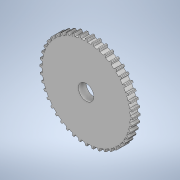
# Autodesk Inventor part: Part14
Saved by Autodesk Inventor 2021 (Build 250183000, 183)
## iProperties
Created: 2022-12-09
Part Number: Part14
Material: Generic
Document SubType Name: Modeling
Designer: user
Density: 1 g/cm^3
Appearance: Default
Author: user
Autodesk Inventor part; units mm, degrees
ref_plane "YZ Plane" through (0, 0, 0) normal (1, 0, 0) x (0, 1, 0)
ref_plane "XZ Plane" through (0, 0, 0) normal (0, 1, 0) x (-1, 0, 0)
ref_plane "XY Plane" through (0, 0, 0) normal (0, 0, 1) x (1, 0, 0)
sketch "Sketch1" plane through (0, 0, 0) normal (0, 0, 1) x (1, 0, 0)
  circle A0 centre (0, 0) radius 20
  arc A1 (-3.5207, 113.9456) -> (-12.7313, 113.2869) centre (0, 0) ccw
  arc A2 (12.7313, 113.2869) -> (3.5207, 113.9456) centre (0, 0) ccw
  arc A3 (-19.701, 112.2848) -> (-28.7241, 110.3219) centre (0, 0) ccw
  arc A4 (-35.4803, 108.3381) -> (-44.1322, 105.1111) centre (0, 0) ccw
  arc A5 (28.7241, 110.3219) -> (19.701, 112.2848) centre (0, 0) ccw
  arc A6 (44.1322, 105.1111) -> (35.4803, 108.3381) centre (0, 0) ccw
  arc A7 (58.6419, 97.7606) -> (50.5373, 102.186) centre (0, 0) ccw
  arc A8 (-50.5373, 102.186) -> (-58.6419, 97.7606) centre (0, 0) ccw
  arc A9 (-64.5655, 93.9537) -> (-71.9577, 88.4199) centre (0, 0) ccw
  arc A10 (-77.2793, 83.8088) -> (-83.8088, 77.2793) centre (0, 0) ccw
  arc A11 (-88.4199, 71.9577) -> (-93.9537, 64.5655) centre (0, 0) ccw
  arc A12 (-97.7606, 58.6419) -> (-102.186, 50.5373) centre (0, 0) ccw
  arc A13 (-105.1111, 44.1322) -> (-108.3381, 35.4803) centre (0, 0) ccw
  arc A14 (-110.3219, 28.7241) -> (-112.2848, 19.701) centre (0, 0) ccw
  arc A15 (-113.2869, 12.7313) -> (-113.9456, 3.5207) centre (0, 0) ccw
  arc A16 (-113.9456, -3.5207) -> (-113.2869, -12.7313) centre (0, 0) ccw
  arc A17 (-112.2848, -19.701) -> (-110.3219, -28.7241) centre (0, 0) ccw
  arc A18 (-108.3381, -35.4803) -> (-105.1111, -44.1322) centre (0, 0) ccw
  arc A19 (-102.186, -50.5373) -> (-97.7606, -58.6419) centre (0, 0) ccw
  arc A20 (-93.9537, -64.5655) -> (-88.4199, -71.9577) centre (0, 0) ccw
  arc A21 (-83.8088, -77.2793) -> (-77.2793, -83.8088) centre (0, 0) ccw
  arc A22 (-71.9577, -88.4199) -> (-64.5655, -93.9537) centre (0, 0) ccw
  arc A23 (-58.6419, -97.7606) -> (-50.5373, -102.186) centre (0, 0) ccw
  arc A24 (-44.1322, -105.1111) -> (-35.4803, -108.3381) centre (0, 0) ccw
  arc A25 (-28.7241, -110.3219) -> (-19.701, -112.2848) centre (0, 0) ccw
  arc A26 (-12.7313, -113.2869) -> (-3.5207, -113.9456) centre (0, 0) ccw
  arc A27 (3.5207, -113.9456) -> (12.7313, -113.2869) centre (0, 0) ccw
  arc A28 (19.701, -112.2848) -> (28.7241, -110.3219) centre (0, 0) ccw
  arc A29 (35.4803, -108.3381) -> (44.1322, -105.1111) centre (0, 0) ccw
  arc A30 (50.5373, -102.186) -> (58.6419, -97.7606) centre (0, 0) ccw
  arc A31 (64.5655, -93.9537) -> (71.9577, -88.4199) centre (0, 0) ccw
  arc A32 (77.2793, -83.8088) -> (83.8088, -77.2793) centre (0, 0) ccw
  arc A33 (88.4199, -71.9577) -> (93.9537, -64.5655) centre (0, 0) ccw
  arc A34 (97.7606, -58.6419) -> (102.186, -50.5373) centre (0, 0) ccw
  arc A35 (105.1111, -44.1322) -> (108.3381, -35.4803) centre (0, 0) ccw
  arc A36 (110.3219, -28.7241) -> (112.2848, -19.701) centre (0, 0) ccw
  arc A37 (113.2869, -12.7313) -> (113.9456, -3.5207) centre (0, 0) ccw
  arc A38 (113.9456, 3.5207) -> (113.2869, 12.7313) centre (0, 0) ccw
  arc A39 (112.2848, 19.701) -> (110.3219, 28.7241) centre (0, 0) ccw
  arc A40 (108.3381, 35.4803) -> (105.1111, 44.1322) centre (0, 0) ccw
  arc A41 (102.186, 50.5373) -> (97.7606, 58.6419) centre (0, 0) ccw
  arc A42 (93.9537, 64.5655) -> (88.4199, 71.9577) centre (0, 0) ccw
  arc A43 (83.8088, 77.2793) -> (77.2793, 83.8088) centre (0, 0) ccw
  arc A44 (71.9577, 88.4199) -> (64.5655, 93.9537) centre (0, 0) ccw
  line L0 (-3.5207, 113.9456) -> (-2.1115, 119.9814)
  line L1 (-2.1115, 119.9814) -> (0, 120)
  line L2 (0, 120) -> (2.1115, 119.9814)
  line L3 (2.1115, 119.9814) -> (3.5207, 113.9456)
  line L4 (-19.701, 112.2848) -> (-19.1651, 118.4597)
  line L5 (-19.1651, 118.4597) -> (-17.0778, 118.7786)
  line L6 (-17.0778, 118.7786) -> (-14.9851, 119.0607)
  line L7 (-14.9851, 119.0607) -> (-12.7313, 113.2869)
  line L8 (-35.4803, 108.3381) -> (-35.8286, 114.5265)
  line L9 (-35.8286, 114.5265) -> (-33.8079, 115.1392)
  line L10 (-33.8079, 115.1392) -> (-31.7767, 115.7162)
  line L11 (-31.7767, 115.7162) -> (-28.7241, 110.3219)
  line L12 (-50.5373, 102.186) -> (-51.7628, 108.2618)
  line L13 (-51.7628, 108.2618) -> (-49.8498, 109.1558)
  line L14 (-49.8498, 109.1558) -> (-47.9214, 110.0161)
  line L15 (-47.9214, 110.0161) -> (-44.1322, 105.1111)
  line L16 (-64.5655, 93.9537) -> (-66.6432, 99.7932)
  line L17 (-66.6432, 99.7932) -> (-64.8769, 100.9504)
  line L18 (-64.8769, 100.9504) -> (-63.0905, 102.0764)
  line L19 (-63.0905, 102.0764) -> (-58.6419, 97.7606)
  line L20 (-77.2793, 83.8088) -> (-80.1669, 89.2932)
  line L21 (-80.1669, 89.2932) -> (-78.5833, 90.6899)
  line L22 (-78.5833, 90.6899) -> (-76.9754, 92.0586)
  line L23 (-76.9754, 92.0586) -> (-71.9577, 88.4199)
  line L24 (-88.4199, 71.9577) -> (-92.0586, 76.9754)
  line L25 (-92.0586, 76.9754) -> (-90.6899, 78.5833)
  line L26 (-90.6899, 78.5833) -> (-89.2932, 80.1669)
  line L27 (-89.2932, 80.1669) -> (-83.8088, 77.2793)
  line L28 (-97.7606, 58.6419) -> (-102.0764, 63.0905)
  line L29 (-102.0764, 63.0905) -> (-100.9504, 64.8769)
  line L30 (-100.9504, 64.8769) -> (-99.7932, 66.6432)
  line L31 (-99.7932, 66.6432) -> (-93.9537, 64.5655)
  line L32 (-105.1111, 44.1322) -> (-110.0161, 47.9214)
  line L33 (-110.0161, 47.9214) -> (-109.1558, 49.8498)
  line L34 (-109.1558, 49.8498) -> (-108.2618, 51.7628)
  line L35 (-108.2618, 51.7628) -> (-102.186, 50.5373)
  line L36 (-110.3219, 28.7241) -> (-115.7162, 31.7767)
  line L37 (-115.7162, 31.7767) -> (-115.1392, 33.8079)
  line L38 (-115.1392, 33.8079) -> (-114.5265, 35.8286)
  line L39 (-114.5265, 35.8286) -> (-108.3381, 35.4803)
  line L40 (-113.2869, 12.7313) -> (-119.0607, 14.9851)
  line L41 (-119.0607, 14.9851) -> (-118.7786, 17.0778)
  line L42 (-118.7786, 17.0778) -> (-118.4597, 19.1651)
  line L43 (-118.4597, 19.1651) -> (-112.2848, 19.701)
  line L44 (-113.9456, -3.5207) -> (-119.9814, -2.1115)
  line L45 (-119.9814, -2.1115) -> (-120, 0)
  line L46 (-120, 0) -> (-119.9814, 2.1115)
  line L47 (-119.9814, 2.1115) -> (-113.9456, 3.5207)
  line L48 (-112.2848, -19.701) -> (-118.4597, -19.1651)
  line L49 (-118.4597, -19.1651) -> (-118.7786, -17.0778)
  line L50 (-118.7786, -17.0778) -> (-119.0607, -14.9851)
  line L51 (-119.0607, -14.9851) -> (-113.2869, -12.7313)
  line L52 (-108.3381, -35.4803) -> (-114.5265, -35.8286)
  line L53 (-114.5265, -35.8286) -> (-115.1392, -33.8079)
  line L54 (-115.1392, -33.8079) -> (-115.7162, -31.7767)
  line L55 (-115.7162, -31.7767) -> (-110.3219, -28.7241)
  line L56 (-102.186, -50.5373) -> (-108.2618, -51.7628)
  line L57 (-108.2618, -51.7628) -> (-109.1558, -49.8498)
  line L58 (-109.1558, -49.8498) -> (-110.0161, -47.9214)
  line L59 (-110.0161, -47.9214) -> (-105.1111, -44.1322)
  line L60 (-93.9537, -64.5655) -> (-99.7932, -66.6432)
  line L61 (-99.7932, -66.6432) -> (-100.9504, -64.8769)
  line L62 (-100.9504, -64.8769) -> (-102.0764, -63.0905)
  line L63 (-102.0764, -63.0905) -> (-97.7606, -58.6419)
  line L64 (-83.8088, -77.2793) -> (-89.2932, -80.1669)
  line L65 (-89.2932, -80.1669) -> (-90.6899, -78.5833)
  line L66 (-90.6899, -78.5833) -> (-92.0586, -76.9754)
  line L67 (-92.0586, -76.9754) -> (-88.4199, -71.9577)
  line L68 (-71.9577, -88.4199) -> (-76.9754, -92.0586)
  line L69 (-76.9754, -92.0586) -> (-78.5833, -90.6899)
  line L70 (-78.5833, -90.6899) -> (-80.1669, -89.2932)
  line L71 (-80.1669, -89.2932) -> (-77.2793, -83.8088)
  line L72 (-58.6419, -97.7606) -> (-63.0905, -102.0764)
  line L73 (-63.0905, -102.0764) -> (-64.8769, -100.9504)
  line L74 (-64.8769, -100.9504) -> (-66.6432, -99.7932)
  line L75 (-66.6432, -99.7932) -> (-64.5655, -93.9537)
  line L76 (-44.1322, -105.1111) -> (-47.9214, -110.0161)
  line L77 (-47.9214, -110.0161) -> (-49.8498, -109.1558)
  line L78 (-49.8498, -109.1558) -> (-51.7628, -108.2618)
  line L79 (-51.7628, -108.2618) -> (-50.5373, -102.186)
  line L80 (-28.7241, -110.3219) -> (-31.7767, -115.7162)
  line L81 (-31.7767, -115.7162) -> (-33.8079, -115.1392)
  line L82 (-33.8079, -115.1392) -> (-35.8286, -114.5265)
  line L83 (-35.8286, -114.5265) -> (-35.4803, -108.3381)
  line L84 (-12.7313, -113.2869) -> (-14.9851, -119.0607)
  line L85 (-14.9851, -119.0607) -> (-17.0778, -118.7786)
  line L86 (-17.0778, -118.7786) -> (-19.1651, -118.4597)
  line L87 (-19.1651, -118.4597) -> (-19.701, -112.2848)
  line L88 (3.5207, -113.9456) -> (2.1115, -119.9814)
  line L89 (2.1115, -119.9814) -> (0, -120)
  line L90 (0, -120) -> (-2.1115, -119.9814)
  line L91 (-2.1115, -119.9814) -> (-3.5207, -113.9456)
  line L92 (19.701, -112.2848) -> (19.1651, -118.4597)
  line L93 (19.1651, -118.4597) -> (17.0778, -118.7786)
  line L94 (17.0778, -118.7786) -> (14.9851, -119.0607)
  line L95 (14.9851, -119.0607) -> (12.7313, -113.2869)
  line L96 (35.4803, -108.3381) -> (35.8286, -114.5265)
  line L97 (35.8286, -114.5265) -> (33.8079, -115.1392)
  line L98 (33.8079, -115.1392) -> (31.7767, -115.7162)
  line L99 (31.7767, -115.7162) -> (28.7241, -110.3219)
  line L100 (50.5373, -102.186) -> (51.7628, -108.2618)
  line L101 (51.7628, -108.2618) -> (49.8498, -109.1558)
  line L102 (49.8498, -109.1558) -> (47.9214, -110.0161)
  line L103 (47.9214, -110.0161) -> (44.1322, -105.1111)
  line L104 (64.5655, -93.9537) -> (66.6432, -99.7932)
  line L105 (66.6432, -99.7932) -> (64.8769, -100.9504)
  line L106 (64.8769, -100.9504) -> (63.0905, -102.0764)
  line L107 (63.0905, -102.0764) -> (58.6419, -97.7606)
  line L108 (77.2793, -83.8088) -> (80.1669, -89.2932)
  line L109 (80.1669, -89.2932) -> (78.5833, -90.6899)
  line L110 (78.5833, -90.6899) -> (76.9754, -92.0586)
  line L111 (76.9754, -92.0586) -> (71.9577, -88.4199)
  line L112 (88.4199, -71.9577) -> (92.0586, -76.9754)
  line L113 (92.0586, -76.9754) -> (90.6899, -78.5833)
  line L114 (90.6899, -78.5833) -> (89.2932, -80.1669)
  line L115 (89.2932, -80.1669) -> (83.8088, -77.2793)
  line L116 (97.7606, -58.6419) -> (102.0764, -63.0905)
  line L117 (102.0764, -63.0905) -> (100.9504, -64.8769)
  line L118 (100.9504, -64.8769) -> (99.7932, -66.6432)
  line L119 (99.7932, -66.6432) -> (93.9537, -64.5655)
  line L120 (105.1111, -44.1322) -> (110.0161, -47.9214)
  line L121 (110.0161, -47.9214) -> (109.1558, -49.8498)
  line L122 (109.1558, -49.8498) -> (108.2618, -51.7628)
  line L123 (108.2618, -51.7628) -> (102.186, -50.5373)
  line L124 (110.3219, -28.7241) -> (115.7162, -31.7767)
  line L125 (115.7162, -31.7767) -> (115.1392, -33.8079)
  line L126 (115.1392, -33.8079) -> (114.5265, -35.8286)
  line L127 (114.5265, -35.8286) -> (108.3381, -35.4803)
  line L128 (113.2869, -12.7313) -> (119.0607, -14.9851)
  line L129 (119.0607, -14.9851) -> (118.7786, -17.0778)
  line L130 (118.7786, -17.0778) -> (118.4597, -19.1651)
  line L131 (118.4597, -19.1651) -> (112.2848, -19.701)
  line L132 (113.9456, 3.5207) -> (119.9814, 2.1115)
  line L133 (119.9814, 2.1115) -> (120, 0)
  line L134 (120, 0) -> (119.9814, -2.1115)
  line L135 (119.9814, -2.1115) -> (113.9456, -3.5207)
  line L136 (112.2848, 19.701) -> (118.4597, 19.1651)
  line L137 (118.4597, 19.1651) -> (118.7786, 17.0778)
  line L138 (118.7786, 17.0778) -> (119.0607, 14.9851)
  line L139 (119.0607, 14.9851) -> (113.2869, 12.7313)
  line L140 (108.3381, 35.4803) -> (114.5265, 35.8286)
  line L141 (114.5265, 35.8286) -> (115.1392, 33.8079)
  line L142 (115.1392, 33.8079) -> (115.7162, 31.7767)
  line L143 (115.7162, 31.7767) -> (110.3219, 28.7241)
  line L144 (102.186, 50.5373) -> (108.2618, 51.7628)
  line L145 (108.2618, 51.7628) -> (109.1558, 49.8498)
  line L146 (109.1558, 49.8498) -> (110.0161, 47.9214)
  line L147 (110.0161, 47.9214) -> (105.1111, 44.1322)
  line L148 (93.9537, 64.5655) -> (99.7932, 66.6432)
  line L149 (99.7932, 66.6432) -> (100.9504, 64.8769)
  line L150 (100.9504, 64.8769) -> (102.0764, 63.0905)
  line L151 (102.0764, 63.0905) -> (97.7606, 58.6419)
  line L152 (83.8088, 77.2793) -> (89.2932, 80.1669)
  line L153 (89.2932, 80.1669) -> (90.6899, 78.5833)
  line L154 (90.6899, 78.5833) -> (92.0586, 76.9754)
  line L155 (92.0586, 76.9754) -> (88.4199, 71.9577)
  line L156 (71.9577, 88.4199) -> (76.9754, 92.0586)
  line L157 (76.9754, 92.0586) -> (78.5833, 90.6899)
  line L158 (78.5833, 90.6899) -> (80.1669, 89.2932)
  line L159 (80.1669, 89.2932) -> (77.2793, 83.8088)
  line L160 (58.6419, 97.7606) -> (63.0905, 102.0764)
  line L161 (63.0905, 102.0764) -> (64.8769, 100.9504)
  line L162 (64.8769, 100.9504) -> (66.6432, 99.7932)
  line L163 (66.6432, 99.7932) -> (64.5655, 93.9537)
  line L164 (44.1322, 105.1111) -> (47.9214, 110.0161)
  line L165 (47.9214, 110.0161) -> (49.8498, 109.1558)
  line L166 (49.8498, 109.1558) -> (51.7628, 108.2618)
  line L167 (51.7628, 108.2618) -> (50.5373, 102.186)
  line L168 (28.7241, 110.3219) -> (31.7767, 115.7162)
  line L169 (31.7767, 115.7162) -> (33.8079, 115.1392)
  line L170 (33.8079, 115.1392) -> (35.8286, 114.5265)
  line L171 (35.8286, 114.5265) -> (35.4803, 108.3381)
  line L172 (12.7313, 113.2869) -> (14.9851, 119.0607)
  line L173 (14.9851, 119.0607) -> (17.0778, 118.7786)
  line L174 (17.0778, 118.7786) -> (19.1651, 118.4597)
  line L175 (19.1651, 118.4597) -> (19.701, 112.2848)
  point P0 (-3.5207, 113.9456)
  point P1 (-12.7313, 113.2869)
  point P2 (-19.701, 112.2848)
  point P3 (-28.7241, 110.3219)
  point P4 (-35.4803, 108.3381)
  point P5 (-44.1322, 105.1111)
  point P6 (-50.5373, 102.186)
  point P7 (-58.6419, 97.7606)
  point P8 (-64.5655, 93.9537)
  point P9 (-71.9577, 88.4199)
  point P10 (-77.2793, 83.8088)
  point P11 (-83.8088, 77.2793)
  point P12 (-88.4199, 71.9577)
  point P13 (-93.9537, 64.5655)
  point P14 (-97.7606, 58.6419)
  point P15 (-102.186, 50.5373)
  point P16 (-108.3381, 35.4803)
  point P17 (-110.3219, 28.7241)
  point P18 (-112.2848, 19.701)
  point P19 (-113.2869, 12.7313)
  point P20 (-113.9456, 3.5207)
  point P21 (-113.9456, -3.5207)
  point P22 (-113.2869, -12.7313)
  point P23 (-112.2848, -19.701)
  point P24 (-110.3219, -28.7241)
  point P25 (-108.3381, -35.4803)
  point P26 (-105.1111, -44.1322)
  point P27 (-102.186, -50.5373)
  point P28 (-97.7606, -58.6419)
  point P29 (-93.9537, -64.5655)
  point P30 (-88.4199, -71.9577)
  point P31 (-83.8088, -77.2793)
  point P32 (-77.2793, -83.8088)
  point P33 (-71.9577, -88.4199)
  point P34 (-64.5655, -93.9537)
  point P35 (-58.6419, -97.7606)
  point P36 (-50.5373, -102.186)
  point P37 (-44.1322, -105.1111)
  point P38 (-35.4803, -108.3381)
  point P39 (-28.7241, -110.3219)
  point P40 (-19.701, -112.2848)
  point P41 (-12.7313, -113.2869)
  point P42 (-3.5207, -113.9456)
  point P43 (3.5207, -113.9456)
  point P44 (12.7313, -113.2869)
  point P45 (19.701, -112.2848)
  point P46 (28.7241, -110.3219)
  point P47 (35.4803, -108.3381)
  point P48 (44.1322, -105.1111)
  point P49 (50.5373, -102.186)
  point P50 (58.6419, -97.7606)
  point P51 (64.5655, -93.9537)
  point P52 (71.9577, -88.4199)
  point P53 (77.2793, -83.8088)
  point P54 (83.8088, -77.2793)
  point P55 (88.4199, -71.9577)
  point P56 (93.9537, -64.5655)
  point P57 (97.7606, -58.6419)
  point P58 (102.186, -50.5373)
  point P59 (108.3381, -35.4803)
  point P60 (110.3219, -28.7241)
  point P61 (112.2848, -19.701)
  point P62 (113.2869, -12.7313)
  point P63 (113.9456, -3.5207)
  point P64 (113.9456, 3.5207)
  point P65 (113.2869, 12.7313)
  point P66 (112.2848, 19.701)
  point P67 (110.3219, 28.7241)
  point P68 (108.3381, 35.4803)
  point P69 (105.1111, 44.1322)
  point P70 (102.186, 50.5373)
  point P71 (97.7606, 58.6419)
  point P72 (93.9537, 64.5655)
  point P73 (88.4199, 71.9577)
  point P74 (83.8088, 77.2793)
  point P75 (71.9577, 88.4199)
  point P76 (64.5655, 93.9537)
  point P77 (58.6419, 97.7606)
  point P78 (50.5373, 102.186)
  point P79 (44.1322, 105.1111)
  point P80 (35.4803, 108.3381)
  point P81 (28.7241, 110.3219)
  point P82 (19.701, 112.2848)
  point P83 (12.7313, 113.2869)
  point P84 (3.5207, 113.9456)
  constraints: 352 end point, 88 point on circle, 45 centre point
extrude "Extrusion1" add sketch "Sketch1" along normal blind 20
body "Solid1"
